Autodesk Fusion 360 part; units mm, degrees
(part 2 of 2)
  line L614 (8.125, -7.0833) -> (8.125, -6.875)
  line L615 (8.125, -6.875) -> (7.7083, -6.875)
  line L616 (7.7083, -6.875) -> (7.7083, -7.0833)
  line L617 (7.7083, -7.0833) -> (7.5, -7.0833)
  line L618 (7.5, -7.0833) -> (7.5, -7.2917)
  line L619 (7.5, -7.2917) -> (7.2917, -7.2917)
  line L620 (7.2917, -7.2917) -> (7.2917, -9.7917)
  line L621 (7.2917, -9.7917) -> (6.875, -9.7917)
  line L622 (6.875, -9.7917) -> (6.875, -7.2917)
  line L623 (6.875, -7.2917) -> (7.0833, -7.2917)
  line L624 (7.0833, -7.2917) -> (7.0833, -7.0833)
  line L625 (7.0833, -7.0833) -> (7.2917, -7.0833)
  line L626 (7.2917, -7.0833) -> (7.2917, -6.875)
  line L627 (7.2917, -6.875) -> (7.5, -6.875)
  line L628 (7.5, -6.875) -> (7.5, -6.6667)
  line L629 (7.5, -6.6667) -> (7.7083, -6.6667)
  line L630 (7.7083, -6.6667) -> (7.7083, -6.4583)
  line L631 (7.7083, -6.4583) -> (8.125, -6.4583)
  line L632 (13.3333, -6.4583) -> (13.3333, -6.875)
  line L633 (13.3333, -6.875) -> (11.875, -6.875)
  line L634 (11.875, -6.875) -> (11.875, -7.9167)
  line L635 (11.875, -7.9167) -> (12.5, -7.9167)
  line L636 (12.5, -7.9167) -> (12.5, -8.3333)
  line L637 (12.5, -8.3333) -> (11.875, -8.3333)
  line L638 (11.875, -8.3333) -> (11.875, -9.375)
  line L639 (11.875, -9.375) -> (13.3333, -9.375)
  line L640 (13.3333, -9.375) -> (13.3333, -9.7917)
  line L641 (13.3333, -9.7917) -> (11.4583, -9.7917)
  line L642 (11.4583, -9.7917) -> (11.4583, -6.4583)
  line L643 (11.4583, -6.4583) -> (13.3333, -6.4583)
  line L644 (17.0833, -6.4583) -> (17.0833, -6.875)
  line L645 (17.0833, -6.875) -> (15.2083, -6.875)
  line L646 (15.2083, -6.875) -> (15.2083, -7.0833)
  line L647 (15.2083, -7.0833) -> (15, -7.0833)
  line L648 (15, -7.0833) -> (15, -7.5)
  line L649 (15, -7.5) -> (15.2083, -7.5)
  line L650 (15.2083, -7.5) -> (15.2083, -7.7083)
  line L651 (15.2083, -7.7083) -> (15.4167, -7.7083)
  line L652 (15.4167, -7.7083) -> (15.4167, -7.9167)
  line L653 (15.4167, -7.9167) -> (16.4583, -7.9167)
  line L654 (16.4583, -7.9167) -> (16.4583, -8.3333)
  line L655 (16.4583, -8.3333) -> (16.6667, -8.3333)
  line L656 (16.6667, -8.3333) -> (16.6667, -8.5417)
  line L657 (16.6667, -8.5417) -> (16.875, -8.5417)
  line L658 (16.875, -8.5417) -> (16.875, -8.75)
  line L659 (16.875, -8.75) -> (17.0833, -8.75)
  line L660 (17.0833, -8.75) -> (17.0833, -9.1667)
  line L661 (17.0833, -9.1667) -> (16.875, -9.1667)
  line L662 (16.875, -9.1667) -> (16.875, -9.375)
  line L663 (16.875, -9.375) -> (16.6667, -9.375)
  line L664 (16.6667, -9.375) -> (16.6667, -9.5833)
  line L665 (16.6667, -9.5833) -> (16.4583, -9.5833)
  line L666 (16.4583, -9.5833) -> (16.4583, -9.7917)
  line L667 (16.4583, -9.7917) -> (14.5833, -9.7917)
  line L668 (14.5833, -9.7917) -> (14.5833, -9.375)
  line L669 (14.5833, -9.375) -> (16.4583, -9.375)
  line L670 (16.4583, -9.375) -> (16.4583, -9.1667)
  line L671 (16.4583, -9.1667) -> (16.6667, -9.1667)
  line L672 (16.6667, -9.1667) -> (16.6667, -8.75)
  line L673 (16.6667, -8.75) -> (16.4583, -8.75)
  line L674 (16.4583, -8.75) -> (16.4583, -8.5417)
  line L675 (16.4583, -8.5417) -> (16.25, -8.5417)
  line L676 (16.25, -8.5417) -> (16.25, -8.3333)
  line L677 (16.25, -8.3333) -> (15.4167, -8.3333)
  line L678 (15.4167, -8.3333) -> (15.4167, -8.125)
  line L679 (15.4167, -8.125) -> (15.2083, -8.125)
  line L680 (15.2083, -8.125) -> (15.2083, -7.9167)
  line L681 (15.2083, -7.9167) -> (15, -7.9167)
  line L682 (15, -7.9167) -> (15, -7.7083)
  line L683 (15, -7.7083) -> (14.7917, -7.7083)
  line L684 (14.7917, -7.7083) -> (14.7917, -7.5)
  line L685 (14.7917, -7.5) -> (14.5833, -7.5)
  line L686 (14.5833, -7.5) -> (14.5833, -7.0833)
  line L687 (14.5833, -7.0833) -> (14.7917, -7.0833)
  line L688 (14.7917, -7.0833) -> (14.7917, -6.875)
  line L689 (14.7917, -6.875) -> (15, -6.875)
  line L690 (15, -6.875) -> (15, -6.6667)
  line L691 (15, -6.6667) -> (15.2083, -6.6667)
  line L692 (15.2083, -6.6667) -> (15.2083, -6.4583)
  line L693 (15.2083, -6.4583) -> (17.0833, -6.4583)
  line L694 (4.7917, -6.875) -> (4.7917, -7.0833)
  line L695 (4.7917, -7.0833) -> (4.5833, -7.0833)
  line L696 (4.5833, -7.0833) -> (4.5833, -7.2917)
  line L697 (4.5833, -7.2917) -> (4.375, -7.2917)
  line L698 (4.375, -7.2917) -> (4.375, -8.75)
  line L699 (4.375, -8.75) -> (5.4167, -8.75)
  line L700 (5.4167, -8.75) -> (5.4167, -7.2917)
  line L701 (5.4167, -7.2917) -> (5.2083, -7.2917)
  line L702 (5.2083, -7.2917) -> (5.2083, -7.0833)
  line L703 (5.2083, -7.0833) -> (5, -7.0833)
  line L704 (5, -7.0833) -> (5, -6.875)
  line L705 (5, -6.875) -> (4.7917, -6.875)
  line L706 (5, -7.2917) -> (5, -7.5)
  line L707 (5, -7.5) -> (5.2083, -7.5)
  line L708 (5.2083, -7.5) -> (5.2083, -8.5417)
  line L709 (5.2083, -8.5417) -> (4.5833, -8.5417)
  line L710 (4.5833, -8.5417) -> (4.5833, -7.5)
  line L711 (4.5833, -7.5) -> (4.7917, -7.5)
  line L712 (4.7917, -7.5) -> (4.7917, -7.2917)
  line L713 (4.7917, -7.2917) -> (5, -7.2917)
extrude "Extrude35" add sketch "Sketch16" along normal blind 1 separate body contours L20 L21 L22 L23 L24 L25 L26 L27 L28 L29 L30 L31 L32 L33 L34 L35 L36 L37 L38 L39 | L40 L41 L42 L43 L44 L45 L46 L47 L48 L49 L50 L51 L52 L53 L54 L55 L56 L57 L58 L59 L60 L61 L62 L63 L64 L65 L66 L67 L68 L69 L70 L71 L72 L73 L74 L75 L76 L77 L78 L79 L80 L81 L82 L83 L84 L85 L86 L87 L88 L89 L90 L91 L92 L93 L94 L95 | L96 L97 L98 L99 L100 L101 L102 L103 L104 L105 L106 L107 L108 L109 L110 L111 L112 L113 L114 L115 L116 L117 L118 L119 | L120 L121 L122 L123 L124 L125 L126 L127 L128 L129 L130 L131 | L132 L133 L134 L135 L136 L137 L138 L139 | L140 L141 L142 L143 L144 L145 L146 L147 L148 L149 L150 L151 L152 L153 L154 L155 L156 L157 | L158 L159 L160 L161 L162 L163 L164 L165 L166 L167 L168 L169 L170 L171 L172 L173 L174 L175 L176 L177 L178 L179 L180 L181 L182 L183 L184 L185 L186 L187 L188 L189 L190 L191 L192 L193 L194 L195 L196 L197 L198 L199 L200 L201 L202 L203 L204 L205 L206 L207 L208 L209 L210 L211 L212 L213 L214 L215 | L216 L217 L218 L219 L220 L221 L222 L223 L224 L225 L226 L227 L228 L229 L230 L231 L232 L233 L234 L235 L236 L237 L238 L239 L240 L241 L242 L243 | L244 L245 L246 L247 L248 L249 L250 L251 L252 L253 L254 L255 | L256 L257 L258 L259 L260 L261 L262 L263 | L264 L265 L266 L267 L268 L269 L270 L271 | L272 L273 L274 L275 L276 L277 L278 L279 | L280 L281 L282 L283 L284 L285 L286 L287 L288 L289 L290 L291 L292 L293 L294 L295 L296 L297 L298 L299 | L300 L301 L302 L303 L304 L305 L306 L307 | L308 L309 L310 L311 L312 L313 L314 L315 L316 L317 L318 L319 L320 L321 L322 L323 L324 L325 L326 L327 | L328 L329 L330 L331 L332 L333 L334 L335 | L336 L337 L338 L339 L340 L341 L342 L343 L344 L345 L346 L347 L348 L349 L350 L351 L352 L353 L354 L355 L356 L357 L358 L359 L360 L361 L362 L363 L364 L365 L366 L367 L368 L369 L370 L371 L372 L373 L374 L375 L376 L377 L378 L379 L380 L381 | L382 L383 L384 L385 L386 L387 L388 L389 L390 L391 L392 L393 L394 L395 L396 L397 L398 L399 L400 L401 L402 L403 L404 L405 | L406 L407 L408 L409 L410 L411 L412 L413 L414 L415 L416 L417 L418 L419 L420 L421 L422 L423 L424 L425 L426 L427 L428 L429 L430 L431 L432 L433 L434 L435 L436 L437 L438 L439 L440 L441 L442 L443 L444 L445 L446 L447 L448 L449 | L450 L451 L452 L453 L454 L455 L456 L457 L458 L459 L460 L461 | L644 L645 L646 L647 L648 L649 L650 L651 L652 L653 L654 L655 L656 L657 L658 L659 L660 L661 L662 L663 L664 L665 L666 L667 L668 L669 L670 L671 L672 L673 L674 L675 L676 L677 L678 L679 L680 L681 L682 L683 L684 L685 L686 L687 L688 L689 L690 L691 L692 L693 | L462 L463 L464 L465 L466 L467 L468 L469 L470 L471 L472 L473 L474 L475 L476 L477 L478 L479 L480 L481 L482 L483 L484 L485 L486 L487 L488 L489 L490 L491 L492 L493 L494 L495 L496 L497 L498 L499 L500 L501 L502 L503 L504 L505 | L506 L507 L508 L509 L510 L511 L512 L513 L514 L515 L516 L517 L518 L519 L520 L521 L522 L523 L524 L525 L526 L527 L528 L529 L530 L531 L532 L533 L534 L535 L536 L537 L538 L539 L540 L541 L542 L543 L544 L545 L546 L547 L548 L549 L550 L551 | L552 L553 L554 L555 L556 L557 L558 L559 L560 L561 L562 L563 L564 L565 L566 L567 L568 L569 L570 L571 L572 L573 L574 L575 | L576 L577 L578 L579 L580 L581 L582 L583 L584 L585 L586 L587 L588 L589 L590 L591 L592 L593 L594 L595 L596 L597 L598 L599 L600 L601 L602 L603 L604 L605 L606 L607 L608 L609 L610 L611 L612 L613 L614 L615 L616 L617 L618 L619 L620 L621 L622 L623 L624 L625 L626 L627 L628 L629 L630 L631 | L632 L633 L634 L635 L636 L637 L638 L639 L640 L641 L642 L643 | L694 L695 L696 L697 L698 L699 L700 L701 L702 L703 L704 L705 | L706 L707 L708 L709 L710 L711 L712 L713 makes body 5 at (15.9028, -16, -6.5278) makes body 6 at (8.8194, -16, -2.7778) makes body 7 at (11.5278, -16, -8.2639) makes body 8 at (5.6944, -16, -4.4444) makes body 9 at (15.625, -16, -2.5694) makes body 10 at (4.7917, -16, -7.7778) makes body 11 at (6.9444, -16, -8.1944) makes body 12 at (12.7083, -16, -3.4028) makes body 13 at (1.9444, -16, -2.0139) makes body 14 at (0.2778, -16, -7.9167)
move_body "Move4" bodies 11 5 8 14 12 13 6 10 7 9 to x (1, 0, 0) y (0, 1, 0) z (0, 0, 1) at (0.7083, 0, 67.6)
move_body "Move5" bodies 14 9 5 10 6 12 11 7 13 8 to x (1, 0, 0) y (0, 1, 0) z (0, 0, 1) at (-2.354, -5, 0)
move_body "Move6" bodies 13 8 6 12 9 5 7 11 10 14 to x (1, 0, 0) y (0, 1, 0) z (0, 0, 1) at (0, 0, -0.05)
move_body "Move7" bodies 13 8 6 12 9 5 7 11 10 14 to x (0, 0, 1) y (0, 1, 0) z (-1, 0, 0) at (68.4043, 0, 55.4457)
extrude "Extrude36" cut 10 faces at (2.8682, -21, 55.7444) (9.1877, -21, 54.0778) (8.6321, -21, 58.5917) (5.2988, -21, 59.4944) (3.6321, -21, 62.6194) (9.0488, -21, 60.7444) (8.8404, -21, 65.3278) (3.0766, -21, 66.0917) (4.9516, -21, 69.425) (7.3821, -21, 69.7028) along direction (0, 1, 0) blind 6 on bodies 5 6 7 8 9 10 11 12 13 14 bodies 3
move_face "MoveFace4" by (0, 0, 0.104) 300 faces at (7.9377, -15.6667, 60.6056) (3.0766, -15, 66.0917) (7.3821, -15, 69.7028) (6.4793, -15.6667, 58.8) (1.4793, -15.6667, 57.6889) (6.0627, -15.6667, 60.3278) (5.7849, -15.6667, 64.8417) (7.521, -15.6667, 68.5222) (8.146, -15.6667, 63.1056) (1.1321, -15.6667, 57.9667) (3.3543, -15.6667, 55.05) (7.3127, -15.6667, 63.7306) (7.5904, -15.6667, 60.8833) (10.8543, -15.6667, 60.7444) (8.6321, -15.6667, 68.3833) (10.021, -15.6667, 61.3) (7.2432, -15.6667, 59.0083) (8.9793, -15.6667, 68.6611) (4.9516, -15, 69.425) (8.6321, -15, 58.5917) (6.2016, -15.6667, 60.2583) (9.2571, -15.6667, 69.0083) (9.0488, -15, 60.7444) (4.2571, -15.6667, 66.925) (1.3404, -15.6667, 57.7583) (9.0488, -15.6667, 62.7583) (7.7293, -15.6667, 64.1472) (3.6321, -15, 62.6194) (3.4932, -15.6667, 60.05) (8.8404, -15, 65.3278) (7.5904, -15.6667, 68.3833) (5.2988, -15, 59.4944) (5.8543, -15.6667, 57.6194) (8.7016, -15.6667, 62.1333) (8.8404, -15.6667, 68.5917) (7.3127, -15.6667, 61.2306) (7.7988, -15.6667, 60.675) (6.0627, -15.6667, 57.8278) (5.4377, -15.6667, 65.3972) (1.5488, -15.6667, 57.55) (1.0627, -15.6667, 58.1056) (1.5488, -15.6667, 67.7583) (8.9793, -15.6667, 70.6056) (7.9377, -15.6667, 66.3694) (3.771, -15.6667, 60.3972) (10.5766, -15.6667, 67.3417) (4.3266, -15.3333, 57.3417) (7.9377, -15.6667, 57.6889) (7.521, -15.6667, 61.0222) (10.021, -15.6667, 58.5917) (9.396, -15.6667, 62.3417) (7.3821, -15.6667, 61.0917) (8.5627, -15.6667, 68.2444) (6.1321, -15.6667, 67.7583) (10.7849, -15.6667, 70.4667) (9.1877, -15.6667, 68.8694) (6.4099, -15.6667, 63.8) (9.7432, -15.6667, 70.05) (10.5766, -15.6667, 56.3) (9.396, -15.6667, 71.0222) (7.7988, -15.6667, 57.7583) (3.2849, -15.6667, 59.8417) (9.0488, -15.6667, 68.8) (5.9932, -15.6667, 60.4667) (6.2016, -15.6667, 64.0083) (7.5904, -15.6667, 57.9667) (6.3404, -15.6667, 58.175) (8.9099, -15.6667, 60.4667) (10.5766, -15.6667, 58.3833) (6.271, -15.6667, 58.0361) (8.3543, -15.6667, 62.8278) (7.3821, -15.6667, 68.5917) (5.7154, -15.6667, 57.55) (6.1321, -15.6667, 57.9667) (8.3543, -15.6667, 61.9944) (7.521, -15.6667, 58.1056) (10.3682, -15.6667, 56.5083) (3.9099, -15.6667, 64.2167) (3.7016, -15.6667, 64.0083) (7.3821, -15.6667, 58.175) (10.7849, -15.6667, 56.0917) (1.896, -15.6667, 65.1194) (7.3127, -15.6667, 58.3139) (8.3543, -15.6667, 61.3694) (10.646, -15.6667, 56.1611) (10.021, -15.6667, 69.425) (3.0766, -15.6667, 65.675) (6.4793, -15.6667, 62.55) (6.4793, -15.6667, 65.8139) (10.8543, -15.6667, 68.9389) (5.646, -15.6667, 57.4111) (8.2154, -15.6667, 61.925) (2.3127, -15.6667, 54.2167) (7.1043, -15.6667, 55.6056) (5.4377, -15.6667, 54.6333) (8.146, -15.6667, 54.9111) (8.2849, -15.6667, 62.9667) (7.3127, -15.6667, 62.2722) (7.521, -15.6667, 63.9389) (10.2293, -15.6667, 54.0778) (7.5904, -15.6667, 54.2167) (10.021, -15.6667, 53.8694) (1.271, -15.6667, 60.1889) (0.8543, -15.6667, 59.2861) (8.9099, -15.6667, 70.4667) (7.6599, -15.6667, 56.0917) (6.271, -15.6667, 60.1194) (0.9932, -15.6667, 63.8) (1.896, -15.6667, 70.5361) (7.6599, -15.6667, 71.0917) (3.9099, -15.6667, 56.0917) (7.521, -15.6667, 59.3556) (1.4099, -15.6667, 64.2167) (7.9377, -15.6667, 69.8417) (7.1043, -15.6667, 61.8556) (3.4932, -15.6667, 64.2167) (1.271, -15.6667, 64.1472) (1.2016, -15.6667, 68.175) (9.6043, -15.6667, 69.9111) (1.4793, -15.6667, 64.3556) (1.0627, -15.6667, 59.9806) (7.1738, -15.6667, 68.8) (7.9377, -15.6667, 59.7722) (1.0627, -15.6667, 63.9389) (5.4377, -15.6667, 67.4806) (10.4377, -15.6667, 54.2861) (1.4099, -15.6667, 60.2583) (10.021, -15.6667, 66.8556) (2.7293, -15.6667, 61.925) (2.3127, -15.6667, 59.4944) (7.7988, -15.6667, 54.0083) (5.4377, -15.6667, 56.6472) (8.2154, -15.6667, 63.3833) (7.7293, -15.6667, 59.5639) (8.3543, -15.6667, 69.3556) (8.2849, -15.6667, 54.8417) (5.9238, -15.6667, 57.7583) (7.9377, -15.6667, 53.9389) (7.1738, -15.6667, 61.3) (0.8543, -15.6667, 70.1194) (9.396, -15.6667, 66.0917) (7.7293, -15.6667, 54.1472) (3.5627, -15.6667, 64.0778) (0.8543, -15.6667, 66.7861) (9.8127, -15.6667, 55.8139) (7.8682, -15.6667, 59.6333) (8.2154, -15.6667, 69.2167) (7.1043, -15.6667, 63.3139) (7.6599, -15.6667, 59.425) (8.5627, -15.6667, 69.9806) (7.1043, -15.6667, 66.5778) (7.2432, -15.6667, 63.5917) (7.1738, -15.6667, 62.7583) (2.3821, -15.6667, 60.675) (1.6877, -15.6667, 60.6056) (1.2016, -15.6667, 64.8417) (7.1043, -15.6667, 58.8) (10.8543, -15.6667, 59.2861) (9.4654, -15.6667, 56.0917) (10.021, -15.6667, 55.4667) (2.7293, -15.6667, 59.9806) (1.4793, -15.6667, 60.3972) (9.4654, -15.6667, 69.8417) (7.6599, -15.6667, 67.3417) (3.3543, -15.6667, 64.2861) (7.2432, -15.6667, 62.1333) (10.5766, -15.6667, 70.675) (9.8821, -15.6667, 55.675) (8.5627, -15.6667, 56.2306) (9.6738, -15.6667, 55.8833) (7.3127, -15.6667, 59.1472) (2.1738, -15.6667, 59.425) (0.8543, -15.6667, 63.175) (8.3543, -15.6667, 63.4528) (7.4516, -15.6667, 63.8) (1.6182, -15.6667, 60.4667) (1.2016, -15.6667, 64.0083) (3.7016, -15.6667, 60.2583) (3.2154, -15.6667, 58.5917) (2.4516, -15.6667, 58.5917) (10.2293, -15.6667, 56.5778) (9.396, -15.6667, 55.5361) (7.1738, -15.6667, 58.3833) (6.4793, -15.6667, 69.425) (8.4932, -15.6667, 69.425) (3.4238, -15.3333, 70.2583) (2.521, -15.6667, 58.4528) (9.8821, -15.6667, 64.425) (9.6043, -15.6667, 56.0222) (8.3543, -15.6667, 65.8833) (8.5627, -15.6667, 66.3) (9.9516, -15.6667, 71.0917) (3.0766, -15.6667, 58.3833) (7.8682, -15.6667, 64.2167) (8.0766, -15.6667, 55.05) (1.2016, -15.6667, 60.05) (7.9377, -15.6667, 55.3972) (3.146, -15.6667, 59.425) (4.9516, -15.3333, 69.0083) (9.1877, -15.6667, 70.8139) (10.646, -15.6667, 70.5361) (9.3266, -15.6667, 70.8833) (7.3821, -15.6667, 62.55) (10.2293, -15.6667, 70.9528) (3.5627, -15.6667, 60.1889) (8.771, -15.6667, 70.3972) (10.8543, -15.6667, 63.8694) (1.5488, -15.6667, 71.0917) (7.9377, -15.6667, 64.3556) (8.8404, -15.6667, 55.2583) (10.3682, -15.6667, 70.8833) (9.1877, -15.6667, 63.5917) (2.2432, -15.6667, 58.8) (5.8543, -15.6667, 60.5361) (3.771, -15.6667, 64.1472) (3.9793, -15.6667, 64.3556) (5.9932, -15.6667, 64.2167) (10.8543, -15.6667, 57.8278) (9.1182, -15.6667, 66.5083) (9.8127, -15.6667, 65.8833) (3.3543, -15.6667, 58.5222) (2.3127, -15.6667, 58.6611) (9.1182, -15.6667, 70.675) (7.521, -15.6667, 54.3556) (1.5488, -15.6667, 54.2167) (9.8821, -15.6667, 59.8417) (1.896, -15.6667, 53.9389) (7.1738, -15.6667, 54.6333) (1.3404, -15.6667, 54.425) (9.1877, -15, 54.0778) (9.7432, -15.6667, 54.8417) (7.1043, -15.6667, 70.3278) (8.3543, -15.6667, 54.7028) (1.896, -15.6667, 67.2028) (7.6599, -15.6667, 64.0083) (2.1043, -15.6667, 59.0083) (7.4516, -15.6667, 59.2167) (1.0627, -15.6667, 54.7722) (9.1877, -15.6667, 54.6333) (10.8543, -15.6667, 55.1194) (7.3821, -15.6667, 54.425) (9.8127, -15.6667, 54.9806) (0.8543, -15.6667, 55.675) (8.6321, -15.6667, 53.8) (2.8682, -15, 55.7444) (1.7571, -15.6667, 54.0083) (0.9238, -15.6667, 54.8417) (1.1321, -15.6667, 54.6333) (9.9516, -15.6667, 55.05) (2.4516, -15.6667, 59.6333) (9.6043, -15.6667, 54.7722) (1.271, -15.6667, 54.5639) (5.7849, -15.6667, 53.8) (10.2988, -15.6667, 54.2167) (8.7016, -15.6667, 70.2583) (1.6877, -15.6667, 54.1472) (6.4793, -15.6667, 54.8417) (7.3127, -15.6667, 54.5639) (8.3543, -15.6667, 65.05) (2.0349, -15.6667, 53.8) (6.1321, -15.6667, 56.925) (10.0904, -15.6667, 54.0083) (7.3127, -15.6667, 62.6889) (0.9238, -15.6667, 58.175) (7.4516, -15.6667, 62.3417) (7.521, -15.6667, 62.4806) (1.4793, -15.6667, 54.3556) (10.5071, -15.6667, 54.425) (2.7293, -15.6667, 64.425) (10.646, -15.6667, 54.4944) (10.7154, -15.6667, 54.6333) (0.9932, -15.6667, 59.8417) (5.2293, -15.6667, 60.675) (8.0071, -15.6667, 68.175) (9.6738, -15.6667, 56.7167) (1.896, -15.6667, 68.4528) (9.396, -15.6667, 69.2861) (8.2849, -15.6667, 61.5083) (7.7293, -15.6667, 60.8139) (10.2988, -15.6667, 68.175) (6.0627, -15.6667, 64.0778) (1.271, -15.6667, 57.8972) (3.3543, -15.6667, 59.9806) (7.7293, -15.6667, 57.8972) (1.6877, -15.6667, 57.4806) (10.4377, -15.6667, 56.3694) (6.4099, -15.6667, 60.05) (10.8543, -15.6667, 65.8139) (3.9793, -15.6667, 60.6056) (6.271, -15.6667, 63.8694) (7.3127, -15.6667, 68.7306) (8.771, -15.6667, 68.4528) (7.7293, -15.6667, 68.3139) (8.146, -15.6667, 61.6472) (8.9099, -15.6667, 57.55) (10.2988, -15.6667, 59.0083) (3.9099, -15.6667, 60.4667) (5.2293, -15.6667, 64.425) (5.8543, -15.6667, 64.2861) (10.4377, -15.6667, 70.7444) on bodies 3
chamfer "Chamfer15" distance 0.5 angle 45 4 faces at (0.3, -6.5833, 44.7) (0.3, -6.5833, 30.2) (13.7, -6.5833, 94.85) (13.7, -6.5833, 80.35) on bodies 1 2
chamfer "Chamfer16" distance 0.5 angle 45 2 faces at (43.0228, 3.1592, 30.2) (43.0228, 3.1592, 44.7) on bodies 4
equation "d15 = 3.6 mm / 2"
equation "d16 = ( 9.2 / 2 ) * 1 mm"
equation "d18 = 1.8 * 2 mm"
equation "d19 = -4.4 mm - ( ( 2.6 * 2 ) * 1 mm ) - 2.4 mm"
equation "d27 = ( 2.6 * 2 ) * 1 mm"
equation "d42 = -29.95 mm + 5 mm"
equation "d58 = ( 4.925 * 2 ) * 1 mm"
equation "d63 = 4.925 mm * 2"
equation "d148 = 65.1 mm + 40 mm"
equation "d154 = 20 mm + 2 mm"
named bodies: "VitaTV Kit Leg", "VitaTV Kit Leg 2", "VitaTV Kit Base", "VitaTV Leg"
